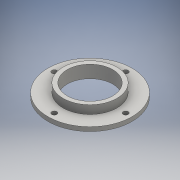
# Autodesk Inventor part: Acople N°1
Saved by Autodesk Inventor 2016 (Build 200138000, 138)
## iProperties
Created: 2017-08-31
Part Number: Acople N°1
Material: Genérico
Document SubType Name: Modeling
Designer: Alumno
Density: 1 g/cm^3
Appearance: Valor por defecto
Author: Alumno
Autodesk Inventor part; units mm, degrees
ref_plane "YZ Plane" through (0, 0, 0) normal (1, 0, 0) x (0, 1, 0)
ref_plane "XZ Plane" through (0, 0, 0) normal (0, 1, 0) x (-1, 0, 0)
ref_plane "XY Plane" through (0, 0, 0) normal (0, 0, 1) x (1, 0, 0)
sketch "Boceto1" plane through (0, 0, 0) normal (0, 0, 1) x (1, 0, 0)
  circle A0 centre (0, 0) radius 16.26
  circle A1 centre (0, 0) radius 19.26
  dimension "d0" = 32.52
  dimension "d1" = 3
  constraints: 2 centre point, 1 coincident
  measures "d0" diameter of A0
  measures "d1" radial gap between concentric circles of A0 A1
extrude "Extrusión1" add sketch "Boceto1" along normal blind 6
sketch "Boceto2" plane through (0, 0, 0) normal (0, 0, -1) x (-1, 0, 0)
  circle A0 centre (0, 0) radius 30
  circle A1 centre (0, 0) radius 16.26 projected
  dimension "d4" = 60
  constraints: 1 centre point, 1 coincident
  measures "d4" diameter of A0
extrude "Extrusión2" add sketch "Boceto2" along normal blind 3
sketch "Boceto3" plane through (0, 0, 0) normal (0, 0, 1) x (1, 0, 0)
  circle A0 centre (0, 0) radius 30 projected
  circle A1 centre (0, 25.5) radius 1.8
  dimension "d7" = 3.6
  dimension "d8" = 25.5
  dimension "d9" = 60
  constraints: 1 centre point
  measures "d7" diameter of A1
  measures "d8" distance of A0.centre A1.centre
  measures "d9" diameter of A0
extrude "Extrusión3" cut sketch "Boceto3" against normal blind 3 contours A1
pattern_circular "Patrón circular1" count 4 over 360 about axis through (0, 0, -10) along (0, 0, 1) of "Extrusión3"
